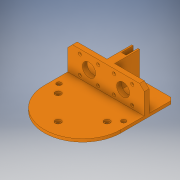
# Autodesk Inventor part: joint_1_base
Saved by Autodesk Inventor 2019 (Build 230136000, 136)
## iProperties
Created: 2019-12-25
Part Number: joint_1_base
Material: Пластик АБС
Document SubType Name: Modeling
Designer: Петров Иван
Density: 1.06 g/cm^3
Appearance: Оранжевый
Author: Петров Иван
Autodesk Inventor part; units mm, degrees
ref_plane "YZ Plane" through (0, 0, 0) normal (1, 0, 0) x (0, 1, 0)
ref_plane "XZ Plane" through (0, 0, 0) normal (0, 1, 0) x (-1, 0, 0)
ref_plane "XY Plane" through (0, 0, 0) normal (0, 0, 1) x (1, 0, 0)
sketch "Эскиз1" plane through (0, 0, 0) normal (0, 1, 0) x (-1, 0, 0)
  circle A0 centre (0, 41.5934) radius 3
  circle A1 centre (41.5934, 0) radius 3
  circle A2 centre (0, -41.5934) radius 3
  arc A3 (-20.609, 31.365) -> (-31.365, 20.609) centre (0, 0) ccw
  arc A4 (-45.7097, 6.2695) -> (-31.365, 20.609) centre (-73.1517, 48.0658) ccw
  arc A5 (-45.7097, 6.2695) -> (-45.7097, -6.2695) centre (-41.5934, 0) ccw
  arc A6 (-31.365, -20.609) -> (-45.7097, -6.2695) centre (-73.1517, -48.0658) ccw
  arc A7 (-31.365, -20.609) -> (-20.609, -31.365) centre (0, 0) ccw
  arc A8 (-6.2695, -45.7097) -> (-20.609, -31.365) centre (-48.0658, -73.1517) ccw
  arc A9 (-6.2695, -45.7097) -> (6.2695, -45.7097) centre (0, -41.5934) ccw
  arc A10 (20.609, -31.365) -> (6.2695, -45.7097) centre (48.0658, -73.1517) ccw
  arc A11 (20.609, -31.365) -> (31.365, -20.609) centre (0, 0) ccw
  arc A12 (45.7097, -6.2695) -> (31.365, -20.609) centre (73.1517, -48.0658) ccw
  arc A13 (45.7097, -6.2695) -> (45.7097, 6.2695) centre (41.5934, 0) ccw
  arc A14 (31.365, 20.609) -> (45.7097, 6.2695) centre (73.1517, 48.0658) ccw
  arc A15 (31.365, 20.609) -> (20.609, 31.365) centre (0, 0) ccw
  arc A16 (6.2695, 45.7097) -> (20.609, 31.365) centre (48.0658, 73.1517) ccw
  arc A17 (6.2695, 45.7097) -> (-6.2695, 45.7097) centre (0, 41.5934) ccw
  arc A18 (-20.609, 31.365) -> (-6.2695, 45.7097) centre (-48.0658, 73.1517) ccw
  circle A19 centre (-41.5934, 0) radius 3
  circle A20 centre (41.5934, 0) radius 3
  circle A21 centre (0, 41.5934) radius 3
  circle A22 centre (-41.5934, 0) radius 3
  circle A23 centre (0, -41.5934) radius 3
  circle A24 centre (0, 0) radius 65
  constraints: 32 point on circle, 25 centre point
extrude "Выдавливание1" add sketch "Эскиз1" along normal blind 5 contours A18 A17 A16 A15 A14 A13 A12 A11 A10 A9 A8 A7 A6 A5 A4 A3 | A24
sketch "Эскиз2" plane through (0, 5, 0) normal (0, 1, 0) x (1, 0, 0)
  circle A0 centre (0, 0) radius 65 projected
  line L0 (65, 0) -> (65, 90)
  line L1 (65, 90) -> (-65, 90)
  line L2 (-65, 90) -> (-65, 0)
  circle A1 centre (41.5934, 0) radius 3 projected
  circle A2 centre (41.5934, 0) radius 3
  circle A3 centre (-41.5934, 0) radius 3 projected
  circle A4 centre (-41.5934, 0) radius 3
  line L3 (-65, 0) -> (-44.5934, 0)
  line L4 (-38.5934, 0) -> (38.5934, 0)
  line L5 (44.5934, 0) -> (65, 0)
  dimension "d2" = 90
  constraints: 12 end point, 4 parallel, 4 point on circle, 3 horizontal, 3 perpendicular, 2 centre point, 2 coincident, 1 concentric, 1 horizontal alignment, 1 other
  measures "d2" distance of L0.end L0.start
extrude "Выдавливание2" add sketch "Эскиз2" against normal blind 5 contours L5 A1 L4 A3 L3 A0 | A0 L2 L1 L0 picked at (0, 22.5961)
chamfer "Фаска1" distance 5 angle 45 2 edges at (65, 2.5, -90) (-65, 2.5, -90)
sketch "Эскиз3" plane through (0, 5, 0) normal (0, 1, 0) x (1, 0, 0)
  line L0 (60, 90) -> (-60, 90)
  line L1 (-8, 80.5) -> (-8, 90)
  line L2 (-40, 47.8) -> (-18, 47.8)
  line L3 (-50, 49.8) -> (-50, 57.5)
  line L4 (-50, 80.5) -> (-50, 90)
  line L5 (-8, 49.8) -> (-8, 57.5)
  line L6 (8, 49.8) -> (8, 57.5)
  line L7 (8, 80.5) -> (8, 90)
  line L8 (50, 49.8) -> (50, 57.5)
  line L9 (50, 80.5) -> (50, 90)
  line L10 (18, 47.8) -> (40, 47.8)
  line L11 (-8, 47.8) -> (-50, 47.8)
  line L12 (-50, 47.8) -> (-50, 90)
  line L13 (-50, 90) -> (-8, 90)
  line L14 (-8, 90) -> (-8, 47.8)
  line L15 (8, 90) -> (50, 90)
  line L16 (50, 90) -> (50, 47.8)
  line L17 (50, 47.8) -> (8, 47.8)
  line L18 (8, 47.8) -> (8, 90)
  line L19 (-65, 0) -> (-65, 85) projected
  line L20 (65, 85) -> (65, 0) projected
  line L21 (-65, 47.8) -> (65, 47.8)
  line L22 (65, 47.8) -> (65, 39.8)
  line L23 (65, 39.8) -> (-65, 39.8)
  line L24 (-65, 39.8) -> (-65, 47.8)
  point P0 (0, 0)
  dimension "d8" = 8
  constraints: 46 end point, 6 parallel, 3 horizontal, 3 perpendicular, 3 point on line
  measures "d8" distance of L21.end L22.end
extrude "Выдавливание3" add sketch "Эскиз3" against normal blind 49 contours L21 L20 L23 L19 L11 L2 L17 L10
sketch "Эскиз5" plane through (-65, 0, -39.8) normal (0, 0, 1) x (1, 0, 0)
  circle A0 centre (94, -21) radius 11.3
  circle A1 centre (36, -21) radius 11
  line L0 (130, 0) -> (130, -44)
  line L1 (130, -44) -> (0, -44)
  point P0 (65, 0)
  dimension "d15" = 22.6
  constraints: 4 end point, 2 centre point
  measures "d15" diameter of A0
extrude "Выдавливание4" cut sketch "Эскиз5" against normal blind 44
sketch "Эскиз6" plane through (-65, 0, -39.8) normal (0, 0, 1) x (1, 0, 0)
  line L0 (111.5, -42) -> (115, -38.5)
  line L1 (115, -38.5) -> (115, -3.5)
  line L2 (115, -3.5) -> (111.5, 0)
  line L3 (111.5, 0) -> (76.5, 0)
  line L4 (76.5, 0) -> (73, -3.5)
  line L5 (73, -3.5) -> (73, -38.5)
  line L6 (73, -38.5) -> (76.5, -42)
  line L7 (76.5, -42) -> (111.5, -42)
  circle A0 centre (94, -21) radius 11.3
  circle A1 centre (109.5, -5.5) radius 1.25
  circle A2 centre (78.5, -5.5) radius 1.25
  circle A3 centre (78.5, -36.5) radius 1.25
  circle A4 centre (109.5, -36.5) radius 1.25
  line L8 (86, -48) -> (88, -48)
  line L9 (88, -41.8) -> (88, -48)
  line L10 (80.5828, -41.8) -> (88, -41.8)
  line L11 (73.2, -34.4172) -> (80.5828, -41.8)
  line L12 (73.2, -7.5828) -> (73.2, -34.4172)
  line L13 (80.5828, -0.2) -> (73.2, -7.5828)
  line L14 (107.4172, -0.2) -> (80.5828, -0.2)
  line L15 (114.8, -7.5828) -> (107.4172, -0.2)
  line L16 (114.8, -34.4172) -> (114.8, -7.5828)
  line L17 (107.4172, -41.8) -> (114.8, -34.4172)
  line L18 (100, -41.8) -> (107.4172, -41.8)
  line L19 (100, -41.8) -> (100, -48)
  line L20 (100, -48) -> (102, -48)
  line L21 (102, -48) -> (102, -42)
  line L22 (102, -42) -> (111.5, -42)
  line L23 (111.5, -42) -> (115, -38.5)
  line L24 (115, -38.5) -> (115, -3.5)
  line L25 (115, -3.5) -> (111.5, 0)
  line L26 (111.5, 0) -> (76.5, 0)
  line L27 (76.5, 0) -> (73, -3.5)
  line L28 (73, -3.5) -> (73, -38.5)
  line L29 (73, -38.5) -> (76.5, -42)
  line L30 (76.5, -42) -> (86, -42)
  line L31 (86, -42) -> (86, -48)
  circle A5 centre (94, -21) radius 11.3 projected
  circle A6 centre (36, -21) radius 11 projected
  line L32 (53.5, -42) -> (57, -38.5)
  line L33 (57, -38.5) -> (57, -3.5)
  line L34 (57, -3.5) -> (53.5, 0)
  line L35 (53.5, 0) -> (18.5, 0)
  line L36 (18.5, 0) -> (15, -3.5)
  line L37 (15, -3.5) -> (15, -38.5)
  line L38 (15, -38.5) -> (18.5, -42)
  line L39 (18.5, -42) -> (53.5, -42)
  circle A7 centre (36, -21) radius 11.3
  circle A8 centre (51.5, -5.5) radius 1.25
  circle A9 centre (20.5, -5.5) radius 1.25
  circle A10 centre (20.5, -36.5) radius 1.25
  circle A11 centre (51.5, -36.5) radius 1.25
  line L40 (28, -48) -> (30, -48)
  line L41 (30, -41.8) -> (30, -48)
  line L42 (22.5828, -41.8) -> (30, -41.8)
  line L43 (15.2, -34.4172) -> (22.5828, -41.8)
  line L44 (15.2, -7.5828) -> (15.2, -34.4172)
  line L45 (22.5828, -0.2) -> (15.2, -7.5828)
  line L46 (49.4172, -0.2) -> (22.5828, -0.2)
  line L47 (56.8, -7.5828) -> (49.4172, -0.2)
  line L48 (56.8, -34.4172) -> (56.8, -7.5828)
  line L49 (49.4172, -41.8) -> (56.8, -34.4172)
  line L50 (42, -41.8) -> (49.4172, -41.8)
  line L51 (42, -41.8) -> (42, -48)
  line L52 (42, -48) -> (44, -48)
  line L53 (44, -48) -> (44, -42)
  line L54 (44, -42) -> (53.5, -42)
  line L55 (53.5, -42) -> (57, -38.5)
  line L56 (57, -38.5) -> (57, -3.5)
  line L57 (57, -3.5) -> (53.5, 0)
  line L58 (53.5, 0) -> (18.5, 0)
  line L59 (18.5, 0) -> (15, -3.5)
  line L60 (15, -3.5) -> (15, -38.5)
  line L61 (15, -38.5) -> (18.5, -42)
  line L62 (18.5, -42) -> (28, -42)
  line L63 (28, -42) -> (28, -48)
  point P0 (65, 0)
  constraints: 128 end point, 10 centre point
extrude "Выдавливание5" cut sketch "Эскиз6" against normal blind 44 contours A1 | A2 | A3 | A4 | A8 | A9 | A10 | A11
chamfer "Фаска3" distance 8 angle 45 2 edges at (65, -44, -43.8) (-65, -44, -43.8)
sketch "Эскиз7" plane through (0, 0, 0) normal (0, -1, 0) x (1, 0, 0)
  circle A0 centre (0, 41.5934) radius 3 projected
  circle A1 centre (0, 41.5934) radius 5
  circle A2 centre (-41.5934, 0) radius 3 projected
  circle A3 centre (-41.5934, 0) radius 5
  circle A4 centre (41.5934, 0) radius 3 projected
  circle A5 centre (41.5934, 0) radius 5
  point P0 (0, 0)
  dimension "d22" = 10
  dimension "d23" = 10
  dimension "d24" = 10
  constraints: 3 centre point, 3 coincident
  measures "d22" diameter of A1
  measures "d23" diameter of A3
  measures "d24" diameter of A5
extrude "Выдавливание6" cut sketch "Эскиз7" against normal blind 3 contours A1 | A2 | A3 | A5
chamfer "Фаска4" distance 1.5 angle 45 8 edges at (43.25, -36.5, -39.8) (12.25, -36.5, -39.8) (12.25, -5.5, -39.8) (43.25, -5.5, -39.8) (-14.75, -36.5, -39.8) (-14.75, -5.5, -39.8) (-45.75, -5.5, -39.8) (-45.75, -36.5, -39.8)
sketch "Эскиз8" plane through (0, 5, 0) normal (0, 1, 0) x (1, 0, 0)
  circle A0 centre (-55, 14.8) radius 4
  circle A1 centre (55, 14.8) radius 4
  line L0 (60, 90) -> (-60, 90)
  point P0 (0, 0)
  constraints: 2 centre point, 2 end point
extrude "Выдавливание7" cut sketch "Эскиз8" against normal through all
sketch "Эскиз9" plane through (65, 0, -47.8) normal (0, 0, -1) x (-1, 0, 0)
  line L0 (122, -44) -> (8, -44) projected
  line L1 (65, -44) -> (65, -22)
  line L2 (71.5, 0) -> (58.5, 0)
  line L3 (58.5, 0) -> (58.5, -44)
  line L4 (58.5, -44) -> (71.5, -44)
  line L5 (71.5, -44) -> (71.5, 0)
  line L6 (71.5, 0) -> (58.5, -44) construction
  line L7 (58.5, 0) -> (71.5, -44) construction
  point P0 (65, 0)
  dimension "d32" = 13
  dimension "d34" = 22
  constraints: 14 end point, 3 midpoint, 2 parallel, 1 horizontal, 1 perpendicular, 1 point on line, 1 vertical
  measures "d32" distance of L4.end L3.end
  measures "d34" distance of L1.start L1.end
extrude "Выдавливание8" add sketch "Эскиз9" along normal up to surface (42.2 mm away)
sketch "Эскиз10" plane through (0, -44, 0) normal (0, -1, 0) x (1, 0, 0)
  line L0 (-6.5, -90) -> (6.5, -90) projected
  line L1 (0, -90) -> (0, -79.9)
  line L2 (-4, -90) -> (4, -90)
  line L3 (4, -90) -> (4, -69.8)
  line L4 (4, -69.8) -> (-4, -69.8)
  line L5 (-4, -69.8) -> (-4, -90)
  line L6 (-4, -90) -> (4, -69.8) construction
  line L7 (4, -90) -> (-4, -69.8) construction
  line L8 (-57, -47.8) -> (-57, -39.8) projected
  line L9 (-57, -47.8) -> (-6.5, -47.8) projected
  line L10 (-6.5, -47.8) -> (-6.5, -90) projected
  line L11 (-6.5, -90) -> (6.5, -90) projected
  line L12 (6.5, -47.8) -> (6.5, -90) projected
  line L13 (6.5, -47.8) -> (57, -47.8) projected
  line L14 (57, -39.8) -> (57, -47.8) projected
  line L15 (57, -39.8) -> (-57, -39.8) projected
  line L16 (-6.5, -47.8) -> (-6.5, -90) projected
  line L17 (-6.5, -47.8) -> (6.5, -47.8)
  line L18 (6.5, -47.8) -> (6.5, -90)
  line L19 (4, -90) -> (6.5, -90)
  line L20 (-4, -90) -> (-6.5, -90)
  line L21 (-6.5, -90) -> (-6.5, -47.8)
  point P0 (0, 0)
  dimension "d37" = 10.1
  dimension "d38" = 8
  dimension "d39" = 20.2
  constraints: 24 end point, 3 equal length, 3 midpoint, 3 perpendicular, 1 horizontal, 1 vertical
  measures "d37" distance of L1.start L1.end
  measures "d38" distance of L4.end L3.end
  measures "d39" distance of L3.end L2.end
extrude "Выдавливание9" cut sketch "Эскиз10" against normal blind 18 contours L5 L4 L3 L0
